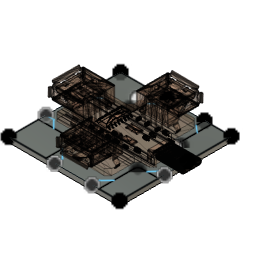
actual usb project v2 (Autodesk Fusion 360 design; units mm, degrees)
Autodesk Fusion 360 part; units mm, degrees
other "Base Mesh Feature1"
other "Body->Comp1"
other "Modify1" in component "OBJ_PCB_usb hub 2.obj"
other "Modify2" in component "OBJ_PCB_usb hub 2.obj"
other "Modify3" in component "OBJ_PCB_usb hub 2.obj"
sketch "Sketch1" plane through (0, 0, 0) normal (0, 0, 1) x (1, 0, 0) in component "top part case"
  line L0 (0, 0) -> (44.562, 0)
  line L1 (44.562, 0) -> (44.562, 44.958)
  line L2 (44.562, 44.958) -> (0, 44.958)
  line L3 (0, 44.958) -> (0, 0)
  dimension "d1" = 44.562
  dimension "d2" = 44.958
  constraint horizontal L0
  constraint vertical L1
  constraint horizontal L2
  constraint vertical L3
  constraint coincident L0.start L3.end
  measures "d1" distance of L0.start L0.end
  measures "d2" distance of L0.start L2.end
other "Modify4" in component "OBJ_PCB_usb hub 2.obj"
other "Scale1" in component "OBJ_PCB_usb hub 2.obj"
other "Modify5" in component "OBJ_PCB_usb hub 2.obj"
other "Scale2" in component "OBJ_PCB_usb hub 2.obj"
other "Modify6" in component "OBJ_PCB_usb hub 2.obj"
other "Scale3" in component "OBJ_PCB_usb hub 2.obj"
other "Modify7" in component "OBJ_PCB_usb hub 2.obj"
other "Scale4" in component "OBJ_PCB_usb hub 2.obj"
other "Modify8" in component "OBJ_PCB_usb hub 2.obj"
extrude "Extrude1" add sketch "Sketch1" along normal blind 2 in component "top part case"
other "Modify9" in component "OBJ_PCB_usb hub 2.obj"
other "Base Mesh Feature1'" in component "top part case"
other "CutPasteMeshes2" in component "OBJ_PCB_usb hub 2.obj"
other "Scale5" in component "OBJ_PCB_usb hub 2.obj"
other "Modify10" in component "OBJ_PCB_usb hub 2.obj"
other "Modify11" in component "OBJ_PCB_usb hub 2.obj"
other "Modify12" in component "OBJ_PCB_usb hub 2.obj"
sketch "Sketch3" plane through (0, 0, 2) normal (0, 0, 1) x (-1, 0, 0) in component "top part case"
  line L0 (0, -44.958) -> (0, 0)
  line L1 (0, 0) -> (-44.562, 0)
  line L2 (-44.562, 0) -> (-44.562, -44.958)
  line L3 (-44.562, -44.958) -> (0, -44.958)
  line L4 (0, 0) -> (-15, 0)
  line L5 (-15, 0) -> (-15, -10.5)
  line L6 (-13.5, -12) -> (0, -12)
  line L7 (0, -12) -> (0, 0)
  arc A0 (-15, -10.5) -> (-13.5, -12) centre (-13.5, -10.5) ccw
  line L8 (0, -44.958) -> (-16.198, -44.958)
  line L9 (-16.198, -44.958) -> (-16.198, -34.048)
  line L10 (-14.698, -32.548) -> (0, -32.548)
  line L11 (0, -32.548) -> (0, -44.958)
  arc A1 (-14.698, -32.548) -> (-16.198, -34.048) centre (-14.698, -34.048) ccw
  line L12 (-44.562, -44.958) -> (-36.395, -44.958)
  line L13 (-36.395, -44.958) -> (-36.395, -31.2)
  line L14 (-37.895, -29.7) -> (-44.562, -29.7)
  line L15 (-44.562, -29.7) -> (-44.562, -44.958)
  arc A2 (-36.395, -31.2) -> (-37.895, -29.7) centre (-37.895, -31.2) ccw
  line L16 (-44.562, 0) -> (-36.315, 0)
  line L17 (-36.315, 0) -> (-36.315, -14.095)
  line L18 (-37.815, -15.595) -> (-44.562, -15.595)
  line L19 (-44.562, -15.595) -> (-44.562, 0)
  arc A3 (-37.815, -15.595) -> (-36.315, -14.095) centre (-37.815, -14.095) ccw
  line L20 (-39.9295, -15.595) -> (-42.0499, -18.058)
  line L21 (-42.0499, -18.058) -> (-44.562, -18.058)
  line L22 (-44.562, -18.058) -> (-44.562, -15.595)
  line L23 (-40.0099, -29.7) -> (-41.9383, -27.4019)
  line L24 (-40.0099, -29.7) -> (-37.0099, -29.7) construction
  line L25 (-41.9383, -27.4019) -> (-44.562, -27.4019)
  line L26 (-44.562, -27.4019) -> (-44.562, -29.7)
  line L27 (-36.395, -39.3091) -> (-33.7138, -41.5589)
  line L28 (-33.7138, -41.5589) -> (-33.7138, -44.958)
  line L29 (-16.198, -39.2549) -> (-18.6729, -41.7298)
  line L30 (-16.198, -39.2549) -> (-12.698, -39.2549) construction
  line L31 (-18.6729, -41.7298) -> (-18.6729, -44.958)
  line L32 (-5.5101, -32.548) -> (-3.5, -30.5)
  line L33 (-3.5, -30.5) -> (0, -30.5)
  line L34 (-6.1, -12) -> (-3.1, -15)
  line L35 (-3.1, -15) -> (0, -15)
  line L36 (-15, -6.6) -> (-18.5, -3.1)
  line L37 (-18.5, -3.1) -> (-18.5, 0)
  line L38 (-36.315, -5.9804) -> (-33.5, -3)
  line L39 (-33.5, -3) -> (-33.5, 0)
  dimension "d11" = 15
  dimension "d12" = 12
  dimension "d13" = 1.5
  dimension "d14" = 16.198
  dimension "d15" = 12.41
  dimension "d16" = 1.5
  dimension "d17" = 8.167
  dimension "d18" = 15.258
  dimension "d19" = 1.5
  dimension "d20" = 8.247
  dimension "d21" = 15.595
  dimension "d22" = 1.5
  dimension "d23" = 3.25
  dimension "d24" = 130
  dimension "d25" = 3
  dimension "d26" = 130
  dimension "d27" = 3.5
  dimension "d28" = 135
  dimension "d29" = 3.5
  constraint horizontal L4
  constraint vertical L5
  constraint horizontal L6
  constraint vertical L7
  constraint coincident L0.end L1.start
  constraint tangent L5 A0
  constraint tangent L6 A0
  constraint horizontal L8
  constraint vertical L9
  constraint horizontal L10
  constraint vertical L11
  constraint coincident L0.start L3.end
  constraint tangent L9 A1
  constraint tangent L10 A1
  constraint horizontal L12
  constraint vertical L13
  constraint horizontal L14
  constraint vertical L15
  constraint coincident L2.end L3.start
  constraint tangent L13 A2
  constraint tangent L14 A2
  constraint horizontal L16
  constraint vertical L17
  constraint horizontal L18
  constraint vertical L19
  constraint coincident L1.end L2.start
  constraint tangent L17 A3
  constraint tangent L18 A3
  constraint coincident L18 L20.start
  constraint coincident L2 L21.end
  constraint perpendicular L2 L21
  constraint horizontal L24
  constraint coincident L14 L23.start
  constraint coincident L2 L25.end
  constraint perpendicular L2 L25
  constraint coincident L13 L27.start
  constraint coincident L3 L28.end
  constraint perpendicular L3 L28
  constraint horizontal L30
  constraint coincident L9 L29.start
  constraint coincident L3 L31.end
  constraint perpendicular L3 L31
  constraint coincident L10 L32.start
  constraint coincident L0 L33.end
  constraint perpendicular L0 L33
  constraint coincident L6 L34.start
  constraint coincident L0 L35.end
  constraint perpendicular L0 L35
  constraint coincident L5 L36.start
  constraint parallel L34 L36
  constraint coincident L1 L37.end
  constraint perpendicular L1 L37
  constraint coincident L17 L38.start
  constraint coincident L1 L39.end
  constraint perpendicular L1 L39
  measures "d11" distance of L0.end L4.end
  measures "d12" distance of L0.end L6.end
  measures "d13" radius of A0
  measures "d14" distance of L0.start L8.end
  measures "d15" distance of L0.start L10.end
  measures "d16" radius of A1
  measures "d17" distance of L2.end L12.end
  measures "d18" distance of L2.end L14.end
  measures "d19" radius of A2
  measures "d20" distance of L1.end L16.end
  measures "d21" distance of L1.end L18.end
  measures "d22" radius of A3
  measures "d23" distance of L20.start L20.end
  measures "d24" angle of L23 L24
  measures "d25" distance of L23.start L23.end
  measures "d26" angle of L26 L27
  measures "d27" distance of L27.start L27.end
  measures "d28" angle of L29 L30
  measures "d29" distance of L29.start L29.end
extrude "Extrude2" [rolled back] along distance -2 taper angle 0 in component "top part case"
extrude "Extrude3" [rolled back] along distance -2 taper angle 0 in component "top part case"
extrude "Extrude4" [rolled back] along distance -2 taper angle 0 in component "top part case"
component "OBJ_PCB_usb hub 2.obj" placed x (1, 0, 0) y (0, 1, 0) z (0, 0, 1) at (0, 0, 0)
component "top part case" placed x (1, 0, 0) y (0, 1, 0) z (0, 0, 1) at (0, 0, 0) in component "OBJ_PCB_usb hub 2.obj"
